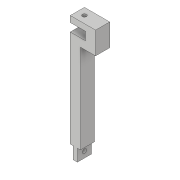
# Autodesk Inventor part: LD_holder_p3
Saved by Autodesk Inventor 2019 (Build 230136000, 136)
## iProperties
Created: 2020-08-30
Part Number: LD_holder_p3
Material: Generic
Document SubType Name: Modeling
Designer: LIU
Density: 1 g/cm^3
Appearance: Default
Author: LIU
Autodesk Inventor part; units mm, degrees
note: some values were not read from the file. Chosen so that the rebuilt part matches the saved one: sketch regions of "Extrusion12".
ref_plane "YZ Plane" through (0, 0, 0) normal (1, 0, 0) x (0, 1, 0)
ref_plane "XZ Plane" through (0, 0, 0) normal (0, 1, 0) x (-1, 0, 0)
ref_plane "XY Plane" through (0, 0, 0) normal (0, 0, 1) x (1, 0, 0)
sketch "Sketch1" plane through (0, 0, 0) normal (0, 1, 0) x (-1, 0, 0)
  line L0 (10, 3.5) -> (-4, 3.5)
  line L1 (-4, 3.5) -> (-4, -3.5)
  line L2 (-4, -3.5) -> (10, -3.5)
  line L3 (10, -3.5) -> (10, 3.5)
  line L4 (12.8, 0) -> (-6.8, 0) projected
  line L5 (0, -4.9) -> (0, 4.9) projected
  circle A0 centre (5, 0) radius 1
  dimension "d13" = 4
  dimension "d14" = 5
  dimension "d15" = 10
  dimension "d16" = 3.5
  dimension "d17" = 3.5
  dimension "d18" = 2
  constraints: 8 end point, 2 parallel, 1 centre point, 1 horizontal, 1 perpendicular, 1 point on line
  measures "d13" distance between parallel lines of L5 L1
  measures "d14" distance from line of A0.centre L5
  measures "d15" distance between parallel lines of L3 L5
  measures "d16" distance between parallel lines of L4 L0
  measures "d17" distance between parallel lines of L2 L4
  measures "d18" diameter of A0
extrude "Extrusion4" add sketch "Sketch1" along normal blind 3 contours L3 L4 A0 L5 L0 | L5 L4 L1 L0 | L3 L2 L5 L4 A0 | L5 L2 L1 L4
sketch "Sketch3" plane through (0, 0, 0) normal (0, -1, 0) x (1, 0, 0)
  line L0 (4, -3.5) -> (-10, -3.5) projected
  line L1 (4, 3.5) -> (4, -3.5) projected
  line L2 (4, 3.5) -> (-1, 3.5)
  line L3 (-1, 3.5) -> (-1, -3.5)
  line L4 (-1, -3.5) -> (4, -3.5)
  line L5 (4, -3.5) -> (4, 3.5)
  point P0 (0, 0)
  dimension "d21" = 5
  constraints: 8 end point, 2 parallel, 1 horizontal, 1 perpendicular, 1 point on line
  measures "d21" distance between parallel lines of L1 L3
extrude "Extrusion5" add sketch "Sketch3" along normal blind 50
sketch "Sketch5" plane through (0, -50, 0) normal (0, -1, 0) x (1, 0, 0)
  line L0 (4, 3.5) -> (-1, 3.5) projected
  line L1 (-1, 3.5) -> (-1, -3.5) projected
  line L2 (-1, -3.5) -> (4, -3.5) projected
  line L3 (4, -3.5) -> (4, 3.5) projected
  line L4 (2.5, 3.5) -> (0.5, 3.5)
  line L5 (0.5, 3.5) -> (0.5, -3.5)
  line L6 (0.5, -3.5) -> (2.5, -3.5)
  line L7 (2.5, -3.5) -> (2.5, 3.5)
  point P0 (0, 0)
  dimension "d29" = 1.5
  dimension "d30" = 1.5
  constraints: 8 end point, 2 parallel, 2 point on line, 1 horizontal, 1 perpendicular
  measures "d29" distance between parallel lines of L3 L7
  measures "d30" distance between parallel lines of L1 L5
extrude "Extrusion7" add sketch "Sketch5" along normal blind 6 contours L7 L2 L5 L0
sketch "Sketch6" plane through (2.5, -50, 3.5) normal (1, 0, 0) x (0, 0, -1)
  circle A0 centre (3.5, -3) radius 1
  line L0 (7, 0) -> (0, 0) projected
  line L1 (0, 0) -> (0, -6) projected
  point P0 (3.5, 50)
  dimension "d34" = 2
  dimension "d35" = 3
  dimension "d36" = 3.5
  constraints: 1 centre point
  measures "d34" diameter of A0
  measures "d35" distance from line of L0 A0.centre
  measures "d36" distance from line of L1 A0.centre
extrude "Extrusion8" cut sketch "Sketch6" against normal through all
sketch "Sketch7" plane through (-1, 0, -3.5) normal (-1, 0, 0) x (0, 0, 1)
  line L0 (0, 0) -> (7, 0) projected
  line L1 (0, 0) -> (0, -50) projected
  line L2 (7, 0) -> (7, -50) projected
  line L3 (0, -4.05) -> (7, -4.05)
  line L4 (7, -4.05) -> (7, -8.05)
  line L5 (7, -8.05) -> (0, -8.05)
  line L6 (0, -8.05) -> (0, -4.05)
  point P0 (3.5, 0)
  dimension "d39" = 4.05
  dimension "d40" = 4
  constraints: 8 end point, 2 parallel, 2 point on line, 1 horizontal, 1 perpendicular
  measures "d39" distance between parallel lines of L0 L3
  measures "d40" distance between parallel lines of L5 L3
extrude "Extrusion9" add sketch "Sketch7" along normal blind 7.5 contours L3 L2 L5 L1
sketch "Sketch9" plane through (-1, -8.05, -3.5) normal (0, -1, 0) x (1, 0, 0)
  line L0 (0, 7) -> (-7.5, 7) projected
  line L1 (-7.5, 0) -> (-7.5, 7) projected
  line L2 (0, 0) -> (-7.5, 0) projected
  line L3 (-7.5, 0) -> (-2.5, 0)
  line L4 (-2.5, 0) -> (-2.5, 7)
  line L5 (-2.5, 7) -> (-7.5, 7)
  line L6 (-7.5, 7) -> (-7.5, 0)
  point P0 (1, 3.5)
  dimension "d43" = 5
  constraints: 8 end point, 2 parallel, 1 horizontal, 1 perpendicular, 1 point on line
  measures "d43" distance between parallel lines of L1 L4
extrude "Extrusion10" add sketch "Sketch9" along normal blind 50
sketch "Sketch10" plane through (-1, -50, -3.5) normal (-1, 0, 0) x (0, 0, 1)
  line L0 (7, 41.95) -> (0, 41.95) projected
  line L1 (0, 41.95) -> (0, 0) projected
  line L2 (7, 0) -> (0, 0) projected
  line L3 (7, 41.95) -> (7, 0) projected
  line L4 (0, 41.95) -> (10.2816, 41.95)
  line L5 (10.2816, 41.95) -> (10.2816, -15.7759)
  line L6 (10.2816, -15.7759) -> (0, -15.7759)
  line L7 (0, -15.7759) -> (0, 41.95)
  point P0 (3.5, 50)
  constraints: 8 end point, 2 parallel, 1 horizontal, 1 perpendicular
extrude "Extrusion11" cut sketch "Sketch10" against normal blind 20
sketch "Sketch11" plane through (-1, -58.05, -3.5) normal (0, -1, 0) x (1, 0, 0)
  line L0 (-2.5, 7) -> (-7.5, 7) projected
  line L1 (-7.5, 7) -> (-7.5, 0) projected
  line L2 (-7.5, 0) -> (-2.5, 0) projected
  line L3 (-2.5, 0) -> (-2.5, 7) projected
  line L4 (-4, 0) -> (-6, 0)
  line L5 (-6, 0) -> (-6, 7)
  line L6 (-6, 7) -> (-4, 7)
  line L7 (-4, 7) -> (-4, 0)
  point P0 (1, 3.5)
  dimension "d48" = 1.5
  dimension "d49" = 1.5
  constraints: 8 end point, 2 parallel, 2 point on line, 1 horizontal, 1 perpendicular
  measures "d48" distance between parallel lines of L3 L7
  measures "d49" distance between parallel lines of L1 L5
extrude "Extrusion12" cut sketch "Sketch11" against normal blind 6 contours L3 L2 L7 L0 | L5 L2 L1 L0
sketch "Sketch12" plane through (-7, -58.05, -3.5) normal (-1, 0, 0) x (0, 0, 1)
  line L0 (7, 6) -> (7, 0) projected
  line L1 (7, 6) -> (0, 6) projected
  circle A0 centre (3.5, 3) radius 1
  point P0 (3.5, 58.05)
  dimension "d52" = 2
  dimension "d53" = 3.5
  dimension "d54" = 3
  constraints: 1 centre point
  measures "d52" diameter of A0
  measures "d53" distance from line of L0 A0.centre
  measures "d54" distance from line of L1 A0.centre
extrude "Extrusion13" cut sketch "Sketch12" against normal through all
thicken "Thicken1" operation add thickness 1 both sides no extend neighbours yes toward (1, 0, 0) faces at (-10, 1, -1.1667)
thicken "Thicken2" operation add thickness 0.5 both sides no extend neighbours yes toward (1, 0, 0) faces at (-9, 1, -1.1667)
body "Solid3"
